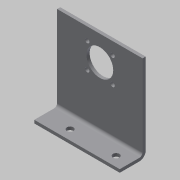
# Autodesk Inventor part: Part157
Saved by Autodesk Inventor 2014 SP1 (Build 180222100, 222)
## iProperties
Created: 2014-12-15
Part Number: Part157
Material: Generic
Document SubType Name: Sheet Metal
Designer: Admin
Density: 1 g/cm^3
Sheet Metal Rule: Default
Appearance: Default
Author: Admin
Autodesk Inventor part; units mm, degrees
ref_plane "YZ Plane" through (0, 0, 0) normal (1, 0, 0) x (0, 1, 0)
ref_plane "XZ Plane" through (0, 0, 0) normal (0, 1, 0) x (-1, 0, 0)
ref_plane "XY Plane" through (0, 0, 0) normal (0, 0, 1) x (1, 0, 0)
sketch "Sketch1" plane through (0, 0, 0) normal (0, 0, 1) x (1, 0, 0)
  line L0 (0, 0) -> (83.6168, 0)
  line L1 (83.6168, 0) -> (83.6168, 85.7504)
  line L2 (83.6168, 85.7504) -> (0, 85.7504)
  line L3 (0, 85.7504) -> (0, 0)
  dimension "d0" = 83.6168
  dimension "d1" = 85.7504
  measures "d0" distance of L2.end L1.end
  measures "d1" distance of L1.end L0.end
extrude "Plate1" add sketch "Sketch1" along normal blind 3.048
sketch "Sketch2" plane through (83.6168, 3.048, 0) normal (0, -1, 0) x (1, 0, 0)
  line L0 (-83.6168, 0) -> (0, 0)
  line L1 (0, 0) -> (0, 25.4)
  line L2 (0, 25.4) -> (-83.6168, 25.4)
  line L3 (-83.6168, 25.4) -> (-83.6168, 0)
  constraints: 6 end point, 1 horizontal, 1 perpendicular, 1 vertical
edge flange "Flange1" height 25.4 angle 90 thickness 3.048 bend radius 3.048 thickness toward (0, -1, 0) relief tear relief width 3.048 relief depth 1.524 edges at (41.8084, 0, 3.048) wall of the first edge with corners at (0, 3.048, 0) (83.6168, 3.048, 0) (83.6168, 3.048, 25.4) (0, 3.048, 25.4)
bend "Bend1"
corner "Corner1"
sketch "Sketch3" plane through (0, 0, 3.048) normal (0, 0, 1) x (1, 0, 0)
  line L0 (83.6168, 85.7504) -> (83.6168, 6.096) projected
  line L1 (0, 0) -> (83.6168, 0) projected
  point P0 (41.8084, 61.2902)
  dimension "d13" = 61.2902
  dimension "d14" = 41.8084
  measures "d13" distance from line of L1 point (41.808, 61.29)
  measures "d14" distance from line of L0 point (41.808, 61.29)
hole "Hole1" at (41.8084, 61.2902, 3.048) direction (0, 0, -1) diameter 26.1112 depth 3.048 tip angle 118
sketch "Sketch4" plane through (0, 0, 3.048) normal (0, 0, 1) x (1, 0, 0)
  circle A0 centre (41.8084, 61.2902) radius 13.0556 projected
  point P0 (0, 0)
  point P1 (29.4386, 73.66)
  point P2 (54.1782, 73.66)
  point P3 (54.1782, 48.9204)
  point P4 (29.4386, 48.9204)
  dimension "d23" = 12.3698
  dimension "d24" = 12.3698
  dimension "d25" = 12.3698
  dimension "d26" = 12.3698
  dimension "d27" = 12.3698
  dimension "d28" = 12.3698
  dimension "d29" = 12.3698
  dimension "d30" = 12.3698
  measures "d23" horizontal distance of A0.centre point (29.439, 73.66)
  measures "d24" horizontal distance of A0.centre point (29.439, 73.66)
  measures "d25" horizontal distance of point (54.178, 73.66) A0.centre
  measures "d26" horizontal distance of A0.centre point (54.178, 73.66)
  measures "d27" horizontal distance of A0.centre point (29.439, 48.92)
  measures "d28" horizontal distance of A0.centre point (29.439, 48.92)
  measures "d29" horizontal distance of point (54.178, 48.92) A0.centre
  measures "d30" horizontal distance of A0.centre point (54.178, 48.92)
hole "Hole2" at (29.4386, 73.66, 3.048) at (54.1782, 73.66, 3.048) at (54.1782, 48.9204, 3.048) at (29.4386, 48.9204, 3.048) direction (0, 0, -1) diameter 4.2926 depth 3.048 tip angle 118
sketch "Sketch5" plane through (0, 3.048, 25.4) normal (0, 1, 0) x (1, 0, 0)
  line L0 (0, 0) -> (0, 19.304) projected
  point P0 (0, 25.4)
  point P1 (25.4, 9.652)
  point P2 (70.4595, 9.652)
  dimension "d39" = 25.4
  measures "d39" distance from line of L0 point (25.4, 9.652)
hole "Hole3" at (25.4, 3.048, 15.748) at (70.4595, 3.048, 15.748) direction (0, -1, 0) diameter 6.35 end through all
equation "\"d20\" = Thickness"
equation "\"d36\" = Thickness"
equation "\"d45\" = Thickness"
equation "\"d3\" = BendReliefWidth"
equation "\"d4\" = BendReliefDepth"
equation "\"d5\" = MinimumRemnant"
equation "\"d6\" = BendRadius"
equation "\"d9\" = BendRadius"
equation "\"d10\" = CornerReliefSize"
equation "\"d11\" = GapSize"
equation "\"d12\" = JacobiRadiusSize"
equation "\"BendRadius\" = Thickness"
equation "\"BendReliefWidth\" = Thickness"
equation "\"BendReliefDepth\" = 0.5 * Thickness"
equation "\"CornerReliefSize\" = 4 * Thickness"
equation "\"MinimumRemnant\" = 2 * Thickness"
equation "\"TransitionRadius\" = BendRadius"
equation "\"JacobiRadiusSize\" = BendRadius"
equation "\"GapSize\" = Thickness"
equation "\"d2\" = BendRadius"
equation "\"Thickness\" = 3.048"
body "Solid1"
